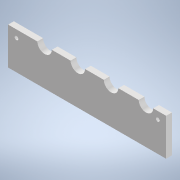
# Autodesk Inventor part: Carcasa_CajaR_Lateral1
Saved by Autodesk Inventor 2022 (Build 260153000, 153)
## iProperties
Created: 2022-02-21
Part Number: Carcasa_CajaR_Lateral1
Material: Generic
Document SubType Name: Modeling
Designer: katha
Density: 1 g/cm^3
Appearance: Default
Author: katha
Autodesk Inventor part; units mm, degrees
ref_plane "YZ Plane" through (0, 0, 0) normal (1, 0, 0) x (0, 1, 0)
ref_plane "XZ Plane" through (0, 0, 0) normal (0, 1, 0) x (-1, 0, 0)
ref_plane "XY Plane" through (0, 0, 0) normal (0, 0, 1) x (1, 0, 0)
sketch "Sketch1" plane through (0, 0, 0) normal (0, 0, 1) x (1, 0, 0)
  circle A0 centre (0, 0) radius 7.5 projected
  circle A1 centre (35.7726, 0) radius 7.5 projected
  line L0 (-37.4458, 2.8981) -> (-34.0994, 2.8981) projected
  line L1 (-39.119, 0) -> (-37.4458, 2.8981) projected
  line L2 (-37.4458, -2.8981) -> (-39.119, 0) projected
  line L3 (-34.0994, -2.8981) -> (-37.4458, -2.8981) projected
  line L4 (-32.4262, 0) -> (-34.0994, -2.8981) projected
  line L5 (-34.0994, 2.8981) -> (-32.4262, 0) projected
  line L6 (71.5994, 2.8981) -> (74.9458, 2.8981) projected
  line L7 (69.9262, 0) -> (71.5994, 2.8981) projected
  line L8 (71.5994, -2.8981) -> (69.9262, 0) projected
  line L9 (74.9458, -2.8981) -> (71.5994, -2.8981) projected
  line L10 (76.619, 0) -> (74.9458, -2.8981) projected
  line L11 (74.9458, 2.8981) -> (76.619, 0) projected
  line L12 (95, 0) -> (95, -40)
  line L13 (95, -40) -> (-75, -40)
  line L14 (-75, -40) -> (-75, 0)
  line L15 (-75, 0) -> (95, 0)
  circle A2 centre (-35.7726, 0) radius 7.5 projected
  circle A3 centre (73.2726, 0) radius 7.5 projected
  circle A4 centre (-35.7726, 0) radius 7.8
  circle A5 centre (0, 0) radius 7.8
  circle A6 centre (35.7726, 0) radius 7.8
  circle A7 centre (73.2726, 0) radius 7.8
  circle A8 centre (86, -8) radius 2
  line L16 (73.2726, 0) -> (73.2726, 6.8626) construction
  line L17 (10, -40) -> (10, -26.4268) construction
  circle A9 centre (-66, -8) radius 2
  point P0 (0, 0)
  point P1 (81.0726, 0)
  point P2 (65.4726, 0)
  point P3 (43.5726, 0)
  point P4 (27.9726, 0)
  point P5 (7.8, 0)
  point P6 (-7.8, 0)
  point P7 (-27.9726, 0)
  point P8 (-43.5726, 0)
  dimension "d2" = 170
  dimension "d3" = 40
  dimension "d4" = 0.3
  dimension "d5" = 0.3
  dimension "d6" = 0.3
  dimension "d7" = 0.3
  dimension "d17" = 4
  dimension "d19" = 8
  dimension "d24" = 9
  constraints: 12 end point, 6 centre point, 2 vertical, 1 coincident, 1 horizontal, 1 midpoint, 1 parallel, 1 perpendicular, 1 symmetric about line, 1 other
  measures "d2" distance of L12.end L13.end
  measures "d3" distance of L12.start L12.end
  measures "d4" radial gap between concentric circles of A2 A4
  measures "d5" radial gap between concentric circles of A0 A5
  measures "d6" radial gap between concentric circles of A1 A6
  measures "d7" radial gap between concentric circles of A3 A7
  measures "d17" diameter of A8
  measures "d19" vertical distance of A8.centre A3.centre
  measures "d24" distance from line of L12 A8.centre
extrude "Extrusion2" add sketch "Sketch1" along normal blind 0.1 and the other way blind 6.1 contours L15 A6 A7 L12 L13 L14 A4 A5
body "Solid2"
